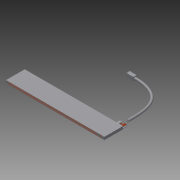
# Autodesk Inventor part: dat4
Saved by Autodesk Inventor 2015 SP1 (Build 190203100, 203)
## iProperties
Created: 2015-12-07
Part Number: dat4
Material: Generic
Document SubType Name: Modeling
Designer: Mihail
Density: 1 g/cm^3
Appearance: Default
Author: Mihail
Autodesk Inventor part; units mm, degrees
ref_plane "YZ Plane" through (0, 0, 0) normal (1, 0, 0) x (0, 1, 0)
sketch "Sketch1" plane through (0, 0, 0) normal (0, 0, 1) x (1, 0, 0)
  line L0 (-105, 20) -> (105, 20)
  line L1 (105, 20) -> (105, -20)
  line L2 (105, -20) -> (-105, -20)
  line L3 (-105, -20) -> (-105, 20)
  line L4 (-105, 20) -> (-100, 20)
  line L5 (-100, 20) -> (-100, -20)
  line L6 (-100, -20) -> (-105, -20)
  line L7 (-105, -20) -> (-105, 20)
  line L8 (-29.7095, -12.3744) -> (-33.2451, -15.9099)
  line L9 (-33.2451, -15.9099) -> (-61.5293, 12.3744)
  line L10 (-61.5293, 12.3744) -> (-57.9938, 15.9099)
  line L11 (-57.9938, 15.9099) -> (-29.7095, -12.3744)
  line L12 (90, 28) -> (95, 28)
  line L13 (95, 28) -> (95, -20)
  line L14 (95, -20) -> (90, -20)
  line L15 (90, -20) -> (90, 28)
  line L16 (100, 28) -> (105, 28)
  line L17 (105, 28) -> (105, -20)
  line L18 (105, -20) -> (100, -20)
  line L19 (100, -20) -> (100, 28)
  line L20 (57.4919, -12.3744) -> (53.9564, -15.9099)
  line L21 (53.9564, -15.9099) -> (25.6721, 12.3744)
  line L22 (25.6721, 12.3744) -> (29.2076, 15.9099)
  line L23 (29.2076, 15.9099) -> (57.4919, -12.3744)
  line L24 (-147, 0) -> (147, 0) projected
  line L25 (0, -29.6) -> (0, 37.6) projected
  point P0 (0, 0)
  point P1 (92.5, -20)
  dimension "d0" = 210
  dimension "d1" = 40
  dimension "d2" = 8
  dimension "d3" = 5
  dimension "d4" = 5
  dimension "d5" = 5
  dimension "d6" = 5
  dimension "d7" = 5
  dimension "d8" = 40
  dimension "d9" = 40
  dimension "d10" = 5
  dimension "d11" = 15.9099
  dimension "d12" = 31.8198
  dimension "d13" = 15.9099
  constraints: 48 end point, 12 parallel, 6 perpendicular, 4 horizontal, 2 collinear, 1 midpoint, 1 point on line, 2 other
  measures "d0" distance of L1.end L2.end
  measures "d1" distance of L0.end L1.end
  measures "d2" distance between parallel lines of L0 L12
  measures "d3" distance of L12.start L12.end
  measures "d4" distance of L16.start L16.end
  measures "d5" distance between parallel lines of L19 L13
  measures "d6" distance between parallel lines of L3 L5
  measures "d7" distance between parallel lines of L11 L9
  measures "d8" distance between parallel lines of L8 L10
  measures "d9" distance between parallel lines of L20 L22
  measures "d10" distance between parallel lines of L23 L21
  measures "d11" distance from line of L24 L10.end
  measures "d12" vertical distance of L8.end L10.end
  measures "d13" distance from line of L24 L23.start
extrude "Extrusion1" add sketch "Sketch1" along normal blind 1 contours L0 L5 L24 L3 | L24 L5 L2 L3 | L15 L12 L13 L0 | L0 L13 L24 L15 | L24 L11 L8 L9 | L9 L10 L11 L24 | L24 L13 L2 L15 | L24 L23 L20 L21 | L21 L22 L23 L24 | L19 L16 L17 L0 | L0 L1 L24 L19 | L24 L1 L2 L19
extrude "Extrusion2" add sketch "Sketch1" against normal blind 1 contours L0 L5 L24 L3 | L0 L25 L24 L11 L10 L9 L5 | L24 L5 L2 L3 | L0 L15 L24 L23 L22 L21 L25 | L24 L9 L8 L11 L25 L2 L5 | L0 L13 L24 L15 | L24 L21 L20 L23 L15 L2 L25 | L24 L11 L8 L9 | L9 L10 L11 L24 | L0 L19 L24 L13 | L24 L13 L2 L15 | L24 L23 L20 L21 | L21 L22 L23 L24 | L0 L1 L24 L19 | L24 L19 L2 L13 | L24 L1 L2 L19
sketch "Sketch2" plane through (0, 0, 1) normal (0, 0, 1) x (1, 0, 0)
  line L0 (-105, -20) -> (-105, 20) projected
  line L1 (-105, 20) -> (105, 20) projected
  line L2 (105, 20) -> (105, -20) projected
  line L3 (105, -20) -> (-105, -20) projected
  point P0 (0, 0)
extrude "Extrusion3" add sketch "Sketch2" along normal blind 1
sketch "Sketch3" plane through (0, 0, 2) normal (0, 0, 1) x (1, 0, 0)
  line L0 (-105, 20) -> (-105, -20) projected
  line L1 (-105, -20) -> (105, -20) projected
  line L2 (105, -20) -> (105, 20) projected
  line L3 (105, 20) -> (-105, 20) projected
  point P0 (0, 0)
extrude "Extrusion4" add sketch "Sketch3" along normal blind 1
sketch "Sketch4" plane through (0, 0, 3) normal (0, 0, 1) x (1, 0, 0)
  line L0 (-105, -20) -> (-105, 20) projected
  line L1 (-105, 20) -> (105, 20) projected
  line L2 (105, 20) -> (105, -20) projected
  line L3 (105, -20) -> (-105, -20) projected
  line L4 (-100, -20) -> (-100, 20) projected
  line L5 (-61.5293, 12.3744) -> (-33.2451, -15.9099) projected
  line L6 (-33.2451, -15.9099) -> (-29.7095, -12.3744) projected
  line L7 (-29.7095, -12.3744) -> (-57.9938, 15.9099) projected
  line L8 (-57.9938, 15.9099) -> (-61.5293, 12.3744) projected
  line L9 (25.6721, 12.3744) -> (53.9564, -15.9099) projected
  line L10 (29.2076, 15.9099) -> (25.6721, 12.3744) projected
  line L11 (57.4919, -12.3744) -> (29.2076, 15.9099) projected
  line L12 (53.9564, -15.9099) -> (57.4919, -12.3744) projected
  line L13 (90, 20) -> (90, -20) projected
  line L14 (90, 28) -> (90, 20) projected
  line L15 (90, 20) -> (95, 20) projected
  line L16 (95, 20) -> (95, 28) projected
  line L17 (95, 28) -> (90, 28) projected
  line L18 (90, 28) -> (90, 20) projected
  line L19 (95, -20) -> (95, 20) projected
  line L20 (-105, -20) -> (105, -20) projected
  line L21 (100, 20) -> (100, -20) projected
  line L22 (105, -20) -> (105, 20) projected
  line L23 (105, 20) -> (105, 28) projected
  line L24 (100, 20) -> (105, 20) projected
  line L25 (105, 20) -> (105, 28) projected
  line L26 (105, 28) -> (100, 28) projected
  line L27 (100, 28) -> (100, 20) projected
  line L28 (105, 20) -> (-105, 20) projected
  line L29 (-105, 20) -> (-105, -20) projected
  line L30 (100, 28) -> (100, -20)
  line L31 (100, -20) -> (105, -20)
  line L32 (105, -20) -> (105, 28)
  line L33 (100, 28) -> (105, 28)
  line L34 (100, 28) -> (100, 20) projected
  point P0 (0, 0)
  constraints: 8 end point, 2 perpendicular, 1 collinear, 1 vertical, 1 other
extrude "Extrusion5" add sketch "Sketch4" along normal blind 1 contours L0 L1 L4 L3 | L13 L1 L19 L3 | L14 L17 L16 L1 | L21 L1 L2 L3 | L27 L26 L23 L1 | L8 L7 L6 L5 | L10 L11 L12 L9
sketch "Sketch5" plane through (0, 0, 4) normal (0, 0, 1) x (1, 0, 0)
  line L0 (-105, -20) -> (-105, 20) projected
  line L1 (-105, 20) -> (105, 20) projected
  line L2 (105, 20) -> (105, -20) projected
  line L3 (105, -20) -> (-105, -20) projected
  point P0 (0, 0)
extrude "Extrusion6" add sketch "Sketch5" along normal blind 1
sketch "Sketch6" plane through (0, 0, 0) normal (0, 0, 1) x (1, 0, 0)
  point P0 (0, 0)
ref_plane "Work Plane1" through (0, 0, 2) normal (0, 0, 1) x (1, 0, 0)
sketch "Sketch7" plane through (0, 0, 2) normal (0, 0, 1) x (1, 0, 0)
  line L0 (100, 20) -> (105, 20) projected
  line L1 (105, 20) -> (105, 28) projected
  line L2 (105, 28) -> (100, 28) projected
  line L3 (100, 28) -> (100, 20) projected
  line L4 (90, 20) -> (95, 20) projected
  line L5 (95, 20) -> (95, 28) projected
  line L6 (95, 28) -> (90, 28) projected
  line L7 (90, 28) -> (90, 20) projected
  line L8 (97.5, 38) -> (97.5, 85.759) construction
  line L9 (97.5, 85.759) -> (92.4337, 108.8931) construction
  line L10 (92.4337, 108.8931) -> (64.4824, 124.1512) construction
  line L11 (64.4824, 124.1512) -> (26.4483, 124.1512) construction
  spline S0 degree 4 poles (97.5, 38) (97.5, 85.759) (92.4337, 108.8931) (64.4824, 124.1512) (26.4483, 124.1512) knots 1 1 1 1 1 2 2 2 2 2
  line L12 (95, 20) -> (95, 28) projected
  line L13 (100, 28) -> (100, 20) projected
  point P0 (0, 0)
  dimension "d27" = 2.5
  dimension "d28" = 10
  constraints: 1 vertical, 3 other
  measures "d27" distance between parallel lines of L5 L8
  measures "d28" distance from line of L6 L8.start
sketch "Sketch9" plane through (0, 0, 3) normal (0, 0, -1) x (-1, 0, 0)
  line L0 (-95, 28) -> (-90, 28) projected
  line L1 (-92.5, 28) -> (-92.5, 33) construction
  line L2 (-92.5, 33) -> (-96.3605, 33) construction
  line L3 (-96.3605, 33) -> (-96.3605, 38) construction
  spline S0 degree 3 poles (-92.5, 28) (-92.5, 33) (-96.3605, 33) (-96.3605, 38) knots 1 1 1 1 2 2 2 2
  point P0 (0, 0)
  dimension "d29" = 5
  dimension "d30" = 10
  constraints: 1 midpoint, 1 perpendicular, 1 vertical, 3 other
  measures "d29" distance between parallel lines of L0 L2
  measures "d30" distance from line of L0 L3.end
sketch "Sketch10" plane through (0, 0, 1) normal (0, 0, 1) x (1, 0, 0)
  spline S0 degree 3 poles (92.5, 28) (92.5, 33) (96.3605, 33) (96.3605, 38) knots 1 1 1 1 2 2 2 2 projected
  point P0 (0, 0)
sketch "Sketch11" plane through (0, 0, 4) normal (0, 0, 1) x (1, 0, 0)
  spline S0 degree 3 poles (92.5, 28) (92.5, 33) (96.3605, 33) (96.3605, 38) knots 1 1 1 1 2 2 2 2 projected
  line L0 (97.5, 38) -> (97.5, 85.759) construction
  line L1 (92.5, 28) -> (92.5, 33) construction
  line L2 (92.5, 33) -> (96.3605, 33) construction
  line L3 (96.3605, 33) -> (96.3605, 38) construction
  line L4 (102.5, 28) -> (102.5, 33) construction
  line L5 (102.5, 33) -> (98.6395, 33) construction
  line L6 (98.6395, 33) -> (98.6395, 38) construction
  line L7 (102.5, 28) -> (102.5, 33) construction
  line L8 (102.5, 33) -> (98.6395, 33) construction
  line L9 (98.6395, 33) -> (98.6395, 38) construction
  spline S1 degree 3 poles (102.5, 28) (102.5, 33) (98.6395, 33) (98.6395, 38) knots 1 1 1 1 2 2 2 2
  point P0 (0, 0)
  constraints: 6 end point, 4 symmetric about line, 3 collinear, 2 coincident, 3 other
sketch "Sketch12" plane through (0, 0, 0) normal (0, 0, -1) x (-1, 0, 0)
  spline S0 degree 3 poles (-102.5, 28) (-102.5, 33) (-98.6395, 33) (-98.6395, 38) knots 1 1 1 1 2 2 2 2 projected
  point P0 (0, 0)
ref_plane "Work Plane3" through (105, 28, 0) normal (0, 0.0995037, -0.9950372) x (-1, 0, 0)
ref_plane "Work Plane4" through (105, 28, 4) normal (0, -0.0995037, -0.9950372) x (-1, 0, 0)
sketch "Sketch13" plane through (105, 28, 0) normal (0, 0.0995037, -0.9950372) x (-1, 0, 0)
  spline S0 degree 3 poles (2.5, 0) (2.5, 4.9752) (6.3605, 4.9752) (6.3605, 9.9504) knots 1 1 1 1 2 2 2 2 projected
  point P0 (105, -27.861)
sketch "Sketch14" plane through (105, 28, 4) normal (0, -0.0995037, -0.9950372) x (-1, 0, 0)
  spline S0 degree 3 poles (2.5, 0) (2.5, 4.9752) (6.3605, 4.9752) (6.3605, 9.9504) knots 1 1 1 1 2 2 2 2 projected
  point P0 (105, -27.463)
ref_plane "Work Plane5" through (97.5, 38, 2) normal (0, 1, 0) x (-1, 0, 0)
sketch "Sketch15" plane through (97.5, 38, 2) normal (0, 1, 0) x (-1, 0, 0)
  circle A0 centre (0, 0) radius 2.5
  circle A1 centre (1.1395, -1) radius 0.4
  circle A2 centre (1.1395, 1) radius 0.4
  circle A3 centre (-1.1395, 1.0099) radius 0.4
  circle A4 centre (-1.1395, -1.0099) radius 0.4
  point P0 (97.5, -2)
  dimension "d31" = 5
  dimension "d32" = 0.8
  dimension "d33" = 0.8
  dimension "d34" = 0.8
  dimension "d35" = 0.8
  constraints: 5 centre point, 5 coincident
  measures "d31" diameter of A0
  measures "d32" diameter of A1
  measures "d33" diameter of A2
  measures "d34" diameter of A3
  measures "d35" diameter of A4
sweep "Sweep1" add profiles "Sketch15" path "Sketch9" path curves S0 contours A2
sweep "Sweep2" add profiles "Sketch15" path "Sketch10" contours A1
sweep "Sweep3" add profiles "Sketch15" path "Sketch14" contours A3
sweep "Sweep4" add profiles "Sketch15" path "Sketch13" contours A4
sweep "Sweep5" add profiles "Sketch15" path "Sketch7" path curves S0 contours A0 | A1 | A2 | A3 | A4
sketch "Sketch16" plane through (0, 0, 2) normal (0, 0, 1) x (1, 0, 0)
  line L0 (26.4483, 126.6512) -> (26.4483, 121.6512) projected
  line L1 (26.4483, 121.6512) -> (26.4483, 120.6512)
  line L2 (26.4483, 120.6512) -> (11.4483, 120.6512)
  line L3 (11.4483, 120.6512) -> (11.4483, 127.6512)
  line L4 (11.4483, 127.6512) -> (14.4483, 128.6512)
  line L5 (14.4483, 128.6512) -> (14.4483, 127.6512)
  line L6 (14.4483, 127.6512) -> (26.4483, 127.6512)
  line L7 (26.4483, 127.6512) -> (26.4483, 126.6512)
  point P0 (0, 0)
  dimension "d46" = 1
  dimension "d47" = 1
  dimension "d48" = 1
  dimension "d49" = 15
  dimension "d50" = 12
  constraints: 14 end point, 4 perpendicular, 1 collinear, 1 parallel, 1 point on line
  measures "d46" distance from line of L6 L0.start
  measures "d47" distance from line of L2 L0.end
  measures "d48" distance of L4.end L5.end
  measures "d49" distance between parallel lines of L1 L3
  measures "d50" distance from line of L7 L5.end
extrude "Extrusion7" add sketch "Sketch16" along normal mid plane 8
sketch "Sketch17" plane through (11.4483, 120.6512, -2) normal (-1, 0, 0) x (0, 0, 1)
  line L0 (0, 0) -> (8, 0) projected
  line L1 (8, 7) -> (8, 0) projected
  line L2 (0, 7) -> (8, 7) projected
  line L3 (0, 0) -> (0, 7) projected
  line L4 (4, 7.876) -> (4, -0.7506)
  line L5 (8, 7) -> (8, 0) projected
  line L6 (1.25, 5.8) -> (2.75, 5.8)
  line L7 (2.75, 5.8) -> (2.75, 4.3)
  line L8 (2.75, 4.3) -> (1.25, 4.3)
  line L9 (1.25, 4.3) -> (1.25, 5.8)
  line L10 (6.75, 5.8) -> (5.25, 5.8)
  line L11 (5.25, 5.8) -> (5.25, 4.3)
  line L12 (5.25, 4.3) -> (6.75, 4.3)
  line L13 (6.75, 4.3) -> (6.75, 5.8)
  point P0 (2, -120.6512)
  dimension "d53" = 4
  dimension "d54" = 1.5
  dimension "d55" = 1.5
  dimension "d56" = 1.2
  dimension "d57" = 4
  constraints: 18 end point, 4 symmetric about line, 3 parallel, 1 horizontal, 1 perpendicular
  measures "d53" distance between parallel lines of L3 L4
  measures "d54" distance of L7.end L8.end
  measures "d55" distance of L6.end L7.end
  measures "d56" distance between parallel lines of L2 L6
  measures "d57" distance between parallel lines of L13 L7
extrude "Extrusion8" cut sketch "Sketch17" against normal blind 12 contours L6 L7 L8 L9 | L13 L12 L11 L10
equation "\"d7\" = d3"
equation "\"d8\" = d1"
equation "\"d9\" = d8"
equation "\"d10\" = d7"
equation "\"d11\" = 0.5 * d12"
equation "\"d13\" = d11"
body "Solid1"
